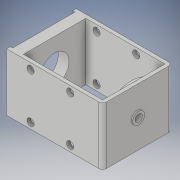
# Autodesk Inventor part: body
Saved by Autodesk Inventor 2017 (Build 210142000, 142)
## iProperties
Created: 2017-01-30
Part Number: body
Material: Generic
Document SubType Name: Modeling
Designer: yul067
Density: 1 g/cm^3
Appearance: Default
Author: yul067
Autodesk Inventor part; units mm, degrees
ref_plane "YZ Plane" through (0, 0, 0) normal (1, 0, 0) x (0, 1, 0)
ref_plane "XZ Plane" through (0, 0, 0) normal (0, 1, 0) x (-1, 0, 0)
ref_plane "XY Plane" through (0, 0, 0) normal (0, 0, 1) x (1, 0, 0)
sketch "Sketch1" plane through (0, 0, 0) normal (0, 0, 1) x (1, 0, 0)
  line L0 (-15.5217, 12.1376) -> (24.4783, 12.1376)
  line L1 (24.4783, 12.1376) -> (24.4783, -11.8624)
  line L2 (24.4783, -11.8624) -> (-15.5217, -11.8624)
  line L3 (-15.5217, -11.8624) -> (-15.5217, 12.1376)
  point P0 (0, 0)
  dimension "d0" = 40
  dimension "d1" = 24
  constraints: 8 end point, 2 parallel, 1 horizontal, 1 perpendicular
  measures "d0" distance of L1.end L2.end
  measures "d1" distance of L0.end L1.end
extrude "Extrusion1" add sketch "Sketch1" along normal blind 29
sketch "Sketch2" plane through (-15.5217, -11.8624, 0) normal (-1, 0, 0) x (0, 0, 1)
  line L0 (0, 0) -> (0, 24) projected
  line L1 (0, 0) -> (29, 0) projected
  line L2 (0, 24) -> (1.5, 24)
  line L3 (1.5, 24) -> (1.5, 0)
  line L4 (1.5, 0) -> (0, 0)
  line L5 (0, 0) -> (0, 24)
  line L6 (0, 24) -> (29, 24) projected
  line L7 (29, 24) -> (27.5, 24)
  line L8 (27.5, 24) -> (27.5, 0)
  line L9 (27.5, 0) -> (29, 0)
  line L10 (29, 0) -> (29, 24)
  line L11 (1.5, 24) -> (27.5, 24)
  line L12 (27.5, 24) -> (27.5, 0)
  line L13 (27.5, 0) -> (1.5, 0)
  line L14 (1.5, 0) -> (1.5, 24)
  point P0 (0, 11.8624)
  dimension "d4" = 1.5
  dimension "d5" = 1.5
  dimension "d6" = 24
  constraints: 24 end point, 6 parallel, 3 horizontal, 3 perpendicular, 1 point on line
  measures "d4" distance of L3.end L4.end
  measures "d5" distance of L9.end L8.end
  measures "d6" distance of L8.end L7.end
extrude "Extrusion2" cut sketch "Sketch2" against normal blind 38.5 contours L3 L6 L8 L1
sketch "Sketch3" plane through (24.4783, -11.8624, 0) normal (1, 0, 0) x (0, 0, -1)
  line L0 (0, 24) -> (-29, 24) projected
  line L1 (0, 24) -> (0, 0) projected
  line L2 (-29, 0) -> (-29, 24) projected
  circle A0 centre (-14.5, 12) radius 1.5
  circle A1 centre (-14.5, 12) radius 2.5
  line L3 (0, 24) -> (-12.574, 13.5939)
  line L4 (-16.426, 10.4061) -> (-29, 0)
  line L5 (-29, 24) -> (-16.426, 13.5939)
  line L6 (-12.574, 10.4061) -> (0, 0)
  point P0 (0, 11.8624)
  dimension "d9" = 3
  dimension "d10" = 5
  constraints: 8 end point, 4 point on circle, 2 centre point, 1 coincident
  measures "d9" diameter of A0
  measures "d10" diameter of A1
extrude "Extrusion3" add sketch "Sketch3" along normal blind 0.5 contours A1
sketch "Sketch4" plane through (24.4783, -11.8624, 0) normal (1, 0, 0) x (0, 0, -1)
  line L0 (0, 24) -> (0, 0) projected
  line L1 (0, 0) -> (-29, 0) projected
  line L2 (0, 24) -> (-29, 0)
  line L3 (0, 24) -> (-29, 24) projected
  line L4 (-29, 24) -> (0, 0)
  circle A0 centre (-14.5, 12) radius 1.5 projected
  circle A1 centre (-14.5, 12) radius 1.5
  point P0 (0, 11.8624)
  dimension "d13" = 3
  constraints: 4 end point, 1 centre point, 1 coincident
  measures "d13" diameter of A1
extrude "Extrusion4" cut sketch "Sketch4" against normal blind 1.5 contours A0 L4 L2 | L2 L4 A0 | A0 L2 L4 | L2 A0 L4
sketch "Sketch5" plane through (-15.5217, -11.8624, 1.5) normal (0, 0, 1) x (1, 0, 0)
  line L0 (0, 24) -> (40, 24) projected
  line L1 (0, 24) -> (1, 24)
  line L2 (1, 24) -> (1, 0)
  line L3 (1, 0) -> (0, 0)
  line L4 (0, 0) -> (0, 24)
  line L5 (1, 24) -> (5.5, 24)
  line L6 (5.5, 24) -> (5.5, 0)
  line L7 (5.5, 0) -> (1, 0)
  line L8 (1, 0) -> (1, 24)
  point P0 (15.5217, 11.8624)
  dimension "d16" = 1
  dimension "d17" = 24
  dimension "d18" = 4.5
  dimension "d19" = 24
  constraints: 16 end point, 4 parallel, 2 horizontal, 2 perpendicular
  measures "d16" distance of L2.end L3.end
  measures "d17" distance of L1.end L2.end
  measures "d18" distance of L6.end L7.end
  measures "d19" distance of L5.end L6.end
extrude "Extrusion5" add sketch "Sketch5" along normal blind 26 contours L0 L6 L7 L2
sketch "Sketch6" plane through (-14.5217, -11.8624, 1.5) normal (-1, 0, 0) x (0, 0, 1)
  line L0 (26, 24) -> (26, 0) projected
  line L1 (-1.5, 24) -> (27.5, 24) projected
  line L2 (26, 0) -> (0, 0) projected
  circle A0 centre (13, 12) radius 6
  line L3 (0, 24) -> (8.5912, 16.0697)
  line L4 (17.4088, 7.9303) -> (26, 0)
  line L5 (26, 24) -> (17.4088, 16.0697)
  line L6 (8.5912, 7.9303) -> (0, 0)
  point P0 (-1.5, 11.8624)
  dimension "d22" = 12
  constraints: 8 end point, 4 point on circle, 1 centre point, 1 point on line
  measures "d22" diameter of A0
extrude "Extrusion6" cut sketch "Sketch6" against normal blind 4.5 contours A0
sketch "Sketch7" plane through (22.9783, -11.8624, 0) normal (-1, 0, 0) x (0, 0, 1)
  line L0 (27.5, 0) -> (1.5, 0) projected
  line L1 (27.5, 24) -> (1.5, 0)
  line L2 (1.5, 0) -> (1.5, 24)
  line L3 (1.5, 24) -> (27.5, 0)
  circle A0 centre (14.5, 12) radius 2.5 projected
  circle A1 centre (14.5, 12) radius 12
  point P0 (0, 11.8624)
  constraints: 6 end point, 1 centre point, 1 coincident, 1 perpendicular
extrude "Extrusion7" add sketch "Sketch7" along normal blind 1 contours A1 L1 A0 L3 | L3 A0 L1 A1 | A1 L3 A0 L1 | A1 L1 A0 L3
fillet "Fillet1" radius 1.5 1 edges at (24.4783, 0.1376, 29)
fillet "Fillet2" radius 1.5 1 edges at (24.4783, 0.1376, 0)
sketch "Sketch8" plane through (0, 0, 29) normal (0, 0, 1) x (1, 0, 0)
  line L0 (-15.5217, -11.8624) -> (-15.5217, 12.1376) projected
  line L1 (-15.5217, 12.1376) -> (-5.5217, 12.1376)
  line L2 (-5.5217, 12.1376) -> (-5.5217, -11.8624)
  line L3 (-5.5217, -11.8624) -> (-15.5217, -11.8624)
  line L4 (-15.5217, -11.8624) -> (-15.5217, 12.1376)
  line L5 (-15.5217, 12.1376) -> (-5.5217, 12.1376)
  line L6 (-7.0217, -9.3624) -> (-15.5217, -9.3624)
  line L7 (-15.5217, -9.3624) -> (-15.5217, 12.1376)
  line L8 (-5.5217, -11.8624) -> (-15.5217, -11.8624)
  line L9 (-15.5217, -11.8624) -> (-15.5217, 9.6376)
  line L10 (-15.5217, 9.6376) -> (-7.0217, 9.6376)
  line L11 (-5.5217, 9.6376) -> (-5.5217, -11.8624)
  circle A0 centre (-5.5217, 9.6376) radius 1.5
  circle A1 centre (-5.5217, -9.3624) radius 1.5
  line L12 (-5.5217, 12.1376) -> (-5.5217, 9.6376)
  line L13 (-5.5217, 8.1376) -> (-5.5217, -9.3624)
  point P0 (0, 0)
  dimension "d35" = 3
  dimension "d29" = 10
  dimension "d30" = 24
  dimension "d31" = 10
  dimension "d32" = 21.5
  dimension "d33" = 21.5
  dimension "d34" = 3
  constraints: 26 end point, 7 parallel, 4 perpendicular, 3 horizontal, 2 coincident, 2 point on circle, 1 centre point, 1 horizontal alignment, 1 point on line, 2 other
  measures "d29" distance of L2.end L3.end
  measures "d30" distance of L1.end L2.end
  measures "d31" distance of L13.end L6.end
  measures "d32" distance of L5.end L13.end
  measures "d33" distance of L8.end L9.end
  measures "d34" diameter of A0
extrude "Extrusion8" cut sketch "Sketch8" against normal blind 29 contours A1 L2 | L2 A1 | A0 L2 | L2 A0
sketch "Sketch9" plane through (0, 0, 29) normal (0, 0, 1) x (1, 0, 0)
  line L0 (-15.5217, 12.1376) -> (-15.5217, -11.8624) projected
  line L1 (-15.5217, 12.1376) -> (10.9783, 12.1376)
  line L2 (10.9783, 12.1376) -> (10.9783, -9.3624)
  line L3 (10.9783, -9.3624) -> (-15.5217, -9.3624)
  line L4 (-15.5217, -9.3624) -> (-15.5217, 12.1376)
  line L5 (10.9783, 12.1376) -> (10.9783, 10.0118)
  circle A0 centre (10.9783, -9.3624) radius 1.5
  circle A1 centre (10.9783, 9.6376) radius 1.5
  point P0 (0, 0)
  dimension "d38" = 26.5
  dimension "d39" = 3
  dimension "d40" = 3
  constraints: 10 end point, 2 centre point, 2 parallel, 2 point on line, 1 coincident, 1 horizontal, 1 perpendicular
  measures "d38" distance of L2.end L3.end
  measures "d39" diameter of A0
  measures "d40" diameter of A1
extrude "Extrusion9" cut sketch "Sketch9" against normal blind 29 contours A0 L2 L3 | L3 L2 A0 | A1 L2 | L2 A1
sketch "Sketch10" plane through (22.9783, 0.1376, 14.5) normal (-1, 0, 0) x (0, 0, 1)
  circle A0 centre (0, 0) radius 1.5 projected
  circle A1 centre (0, 0) radius 2.5
  point P0 (-14.5, -0.1376)
  dimension "d43" = 5
  constraints: 1 centre point, 1 coincident
  measures "d43" diameter of A1
extrude "Extrusion10" add sketch "Sketch10" along normal blind 1
body "Solid1"
